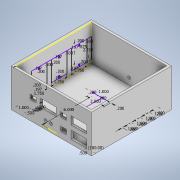
# Autodesk Inventor part: box thin walled
Saved by Autodesk Inventor 2020 (Build 240168000, 168)
## iProperties
Created: 2020-01-13
Part Number: box thin walled
Material: Generic
Document SubType Name: Modeling
Designer: ColinP
Density: 1 g/cm^3
Appearance: Default
Author: ColinP
Autodesk Inventor part; units mm, degrees
ref_plane "YZ Plane" through (0, 0, 0) normal (1, 0, 0) x (0, 1, 0)
ref_plane "XZ Plane" through (0, 0, 0) normal (0, 1, 0) x (-1, 0, 0)
ref_plane "XY Plane" through (0, 0, 0) normal (0, 0, 1) x (1, 0, 0)
sketch "Sketch1" plane through (0, 0, 0) normal (0, 1, 0) x (-1, 0, 0)
  line L0 (0, 0) -> (-114.3, 0)
  line L1 (-114.3, 0) -> (-114.3, -114.3)
  line L2 (-114.3, -114.3) -> (114.3, -114.3)
  line L3 (114.3, -114.3) -> (114.3, 114.3)
  line L4 (114.3, 114.3) -> (-114.3, 114.3)
  line L5 (-114.3, 114.3) -> (-114.3, 0)
  dimension "d0" = 114.3
  dimension "d1" = 114.3
  dimension "d2" = 228.6
  dimension "d3" = 228.6
  dimension "d4" = 90
  constraints: 12 end point, 4 perpendicular, 1 collinear, 1 horizontal, 1 point on line
  measures "d0" distance of L0.start L0.end
  measures "d1" distance of L0.end L1.end
  measures "d2" distance of L1.end L2.end
  measures "d3" distance of L2.end L3.end
  measures "d4" angle of L3 L2
extrude "Extrusion1" add sketch "Sketch1" along normal blind 6.35
sketch "Sketch3" plane through (0, 6.35, 0) normal (0, 1, 0) x (1, 0, 0)
  line L0 (114.3, 114.3) -> (-114.3, 114.3) projected
  line L1 (-114.3, 114.3) -> (-108.2442, 114.3)
  line L2 (-108.2442, 114.3) -> (-108.2442, -114.3)
  line L3 (-108.2442, 114.3) -> (120.3558, 114.3) construction
  line L4 (-108.2442, -114.3) -> (-108.2442, -107.95)
  line L5 (-108.2442, -107.95) -> (107.6558, -107.95)
  line L6 (107.6558, -107.95) -> (107.6558, 107.95)
  line L7 (107.6558, 107.95) -> (-108.2442, 107.95)
  line L8 (-114.3, 114.3) -> (-114.3, -114.3) projected
  line L9 (-114.3, -114.3) -> (114.3, -114.3) projected
  line L10 (114.3, -114.3) -> (114.3, 114.3) projected
  point P0 (0, 0)
  dimension "d19" = 228.6
  dimension "d20" = 90
  dimension "d21" = 6.35
  dimension "d22" = 215.9
  dimension "d23" = 215.9
  constraints: 14 end point, 4 perpendicular, 3 point on line, 1 horizontal, 1 vertical
  measures "d19" distance of L1.end L2.end
  measures "d20" angle of L2 L3
  measures "d21" distance of L2.end L4.end
  measures "d22" distance of L4.end L5.end
  measures "d23" distance of L5.end L6.end
extrude "Extrusion3" add sketch "Sketch3" along normal blind 101.6 contours L10 L9 L2 L5 L6 L7 L0 | L2 L9 L8 L0
sketch "Sketch4" plane through (-114.3, 0, 114.3) normal (0, 0, 1) x (1, 0, 0)
  line L0 (221.9558, 6.35) -> (221.9558, 107.95) projected
  line L1 (221.9558, 107.95) -> (221.9558, 44.45)
  line L2 (221.9558, 6.35) -> (6.0558, 6.35) projected
  line L3 (221.9558, 6.35) -> (221.9558, 12.7)
  line L4 (221.9558, 6.35) -> (221.9558, 107.95) projected
  line L5 (221.9558, 12.7) -> (215.6058, 12.7)
  line L6 (215.6058, 12.7) -> (215.6058, 35.2044)
  line L7 (215.6058, 35.2044) -> (170.597, 35.2044)
  line L8 (170.597, 35.2044) -> (170.597, 12.7)
  line L9 (170.597, 12.7) -> (215.6058, 12.7)
  line L10 (170.597, 12.7) -> (157.897, 12.7)
  line L11 (157.897, 12.7) -> (157.897, 35.2044)
  line L12 (157.897, 35.2044) -> (112.8882, 35.2044)
  line L13 (112.8882, 35.2044) -> (112.8882, 12.7)
  line L14 (112.8882, 12.7) -> (157.897, 12.7)
  line L15 (112.8882, 35.2044) -> (100.1882, 35.2044)
  line L16 (100.1882, 35.2044) -> (100.1882, 12.7)
  line L17 (100.1882, 12.7) -> (55.1794, 12.7)
  line L18 (55.1794, 12.7) -> (55.1794, 35.2044)
  line L19 (55.1794, 35.2044) -> (100.1882, 35.2044)
  line L20 (215.6058, 35.2044) -> (215.6058, 47.9044)
  line L21 (215.6058, 47.9044) -> (170.597, 47.9044)
  line L22 (170.597, 47.9044) -> (170.597, 70.4088)
  line L23 (170.597, 70.4088) -> (215.6058, 70.4088)
  line L24 (215.6058, 70.4088) -> (215.6058, 47.9044)
  line L25 (215.6058, 70.4088) -> (215.6058, 83.1088)
  point P0 (114.3, 0)
  point P1 (215.6058, 105.6132)
  point P2 (170.597, 105.6132)
  point P3 (170.597, 83.1088)
  dimension "d34" = 6.35
  dimension "d35" = 6.35
  dimension "d36" = 22.5044
  dimension "d37" = 45.0088
  dimension "d38" = 12.7
  dimension "d39" = 45.0088
  dimension "d40" = 12.7
  dimension "d41" = 45.0088
  dimension "d44" = 12.7
  dimension "d45" = 22.5044
  dimension "d46" = 12.7
  dimension "d47" = 22.5044
  constraints: 46 end point, 15 point on line, 14 perpendicular, 1 horizontal, 1 vertical
  measures "d34" distance of L0.start L3.end
  measures "d35" distance of L3.end L5.end
  measures "d36" distance of L5.end L6.end
  measures "d37" distance of L6.end L7.end
  measures "d38" distance of L8.end L10.end
  measures "d39" distance of L11.end L12.end
  measures "d40" distance of L12.end L15.end
  measures "d41" distance of L16.end L17.end
  measures "d44" distance of L6.end L20.end
  measures "d45" distance of L21.end L22.end
  measures "d46" distance of L23.end L25.end
  measures "d47" distance of L25.end point (215.606, 105.613)
sketch "Sketch9" plane through (-114.3, 0, 114.3) normal (0, 0, 1) x (1, 0, 0)
  line L0 (170.597, 47.9044) -> (170.597, 70.4088) projected
  line L1 (170.597, 70.4088) -> (170.597, 59.1566)
  line L2 (170.597, 59.1566) -> (157.897, 59.1566)
  line L3 (170.597, 35.0034) -> (170.597, 23.7512)
  line L4 (170.597, 23.7512) -> (157.897, 23.7512)
  line L5 (157.897, 59.1566) -> (157.897, 65.6066)
  line L6 (157.897, 65.6066) -> (141.197, 65.6066)
  line L7 (141.197, 65.6066) -> (141.197, 52.7034)
  line L8 (141.197, 52.7034) -> (157.897, 52.7034)
  line L9 (157.897, 52.7034) -> (157.897, 59.1566)
  line L10 (157.897, 23.7512) -> (157.897, 30.2012)
  line L11 (157.897, 30.2012) -> (141.197, 30.2012)
  line L12 (141.197, 30.2012) -> (141.197, 17.3012)
  line L13 (141.197, 17.3012) -> (157.897, 17.3012)
  line L14 (157.897, 17.3012) -> (157.897, 23.7512)
  point P0 (114.3, 0)
  point P1 (170.597, 105.6132)
  dimension "d64" = 11.2522
  dimension "d65" = 12.7
  dimension "d67" = 11.2522
  dimension "d68" = 12.7
  dimension "d82" = 6.45
  dimension "d83" = 12.9032
  dimension "d84" = 6.45
  dimension "d85" = 12.9
  constraints: 28 end point, 7 perpendicular, 4 point on line, 1 midpoint, 1 vertical
  measures "d64" distance of L0.end L1.end
  measures "d65" distance of L1.end L2.end
  measures "d67" distance of L3.start L3.end
  measures "d68" distance of L3.end L4.end
  measures "d82" distance of L2.end L5.end
  measures "d83" distance of L6.end L7.end
  measures "d84" distance of L4.end L10.end
  measures "d85" distance of L11.end L12.end
extrude "Extrusion4" cut sketch "Sketch4" against normal blind 114.3 contours L9 L8 L7 L6 | L21 L22 L23 L24
extrude "Extrusion6" cut sketch "Sketch9" against normal blind 114.3
sketch "Sketch14" plane through (-108.2442, 6.35, 107.95) normal (1, 0, 0) x (0, 0, -1)
  line L0 (215.9, 0) -> (0, 0) projected
  line L1 (0, 0) -> (0, 101.6) projected
  line L2 (-6.35, 101.6) -> (0, 101.6)
  line L3 (0, 101.6) -> (215.9, 101.6) projected
  line L4 (215.9, 0) -> (215.9, 101.6) projected
  line L5 (215.9, 66.675) -> (215.9, 9.525)
  line L6 (215.9, 66.675) -> (203.2, 66.675)
  line L7 (203.2, 66.675) -> (203.2, 9.525)
  line L8 (203.2, 9.525) -> (158.75, 9.525)
  line L9 (158.75, 9.525) -> (158.75, 66.675)
  line L10 (158.75, 66.675) -> (203.2, 66.675)
  line L11 (158.75, 66.675) -> (146.05, 66.675)
  line L12 (146.05, 66.675) -> (146.05, 9.525)
  line L13 (146.05, 9.525) -> (101.6, 9.525)
  line L14 (101.6, 9.525) -> (101.6, 66.675)
  line L15 (101.6, 66.675) -> (146.05, 66.675)
  line L16 (101.6, 66.675) -> (88.9, 66.675)
  line L17 (88.9, 66.675) -> (88.9, 9.525)
  line L18 (88.9, 9.525) -> (44.45, 9.525)
  line L19 (44.45, 9.525) -> (44.45, 66.675)
  line L20 (44.45, 66.675) -> (88.9, 66.675)
  line L21 (203.2, 66.675) -> (180.975, 66.675)
  line L22 (180.975, 66.675) -> (180.975, 61.675)
  line L23 (180.975, 9.525) -> (180.975, 14.525)
  circle A0 centre (180.975, 61.675) radius 2.54
  circle A1 centre (180.975, 14.525) radius 2.54
  line L24 (123.825, 66.675) -> (123.825, 61.675)
  line L25 (123.825, 9.525) -> (123.825, 14.525)
  circle A2 centre (123.825, 61.675) radius 2.54
  circle A3 centre (123.825, 14.525) radius 2.54
  line L26 (66.675, 66.675) -> (66.675, 61.675)
  line L27 (66.675, 9.525) -> (66.675, 14.525)
  circle A4 centre (66.675, 61.675) radius 2.54
  circle A5 centre (66.675, 14.525) radius 2.54
  point P0 (107.95, -6.35)
  dimension "d123" = 57.15
  dimension "d124" = 12.7
  dimension "d125" = 44.45
  dimension "d126" = 12.7
  dimension "d127" = 44.45
  dimension "d128" = 12.7
  dimension "d129" = 44.45
  dimension "d139" = 22.225
  dimension "d140" = 5
  dimension "d141" = 5
  dimension "d142" = 5.08
  dimension "d143" = 5.08
  dimension "d144" = 5
  dimension "d145" = 5
  dimension "d146" = 5.08
  dimension "d147" = 5.08
  dimension "d148" = 5
  dimension "d149" = 5
  dimension "d150" = 5.08
  dimension "d151" = 5.08
  constraints: 48 end point, 11 perpendicular, 11 point on line, 6 centre point, 6 coincident, 6 midpoint, 5 vertical, 1 collinear, 1 horizontal
  measures "d123" distance of L5.start L5.end
  measures "d124" distance of L5.start L6.end
  measures "d125" distance of L7.end L8.end
  measures "d126" distance of L9.end L11.end
  measures "d127" distance of L12.end L13.end
  measures "d128" distance of L14.end L16.end
  measures "d129" distance of L17.end L18.end
  measures "d139" distance of L6.end L21.end
  measures "d140" distance of L21.end L22.end
  measures "d141" distance of L23.start L23.end
  measures "d142" diameter of A0
  measures "d143" diameter of A1
  measures "d144" distance of L24.start L24.end
  measures "d145" distance of L25.start L25.end
  measures "d146" diameter of A2
  measures "d147" diameter of A3
  measures "d148" distance of L26.start L26.end
  measures "d149" distance of L27.start L27.end
  measures "d150" diameter of A4
  measures "d151" diameter of A5
sketch "Sketch15" plane through (-114.3, 0, 114.3) normal (0, 0, 1) x (1, 0, 0)
  line L0 (141.197, 65.6066) -> (141.197, 52.7034) projected
  line L1 (141.197, 59.155) -> (128.497, 59.155)
  line L2 (128.497, 59.155) -> (128.497, 70.4088)
  line L3 (128.497, 70.4088) -> (128.497, 47.9044)
  line L4 (215.6058, 47.9044) -> (170.597, 47.9044) projected
  line L5 (128.497, 47.9044) -> (83.4882, 47.9044)
  line L6 (83.4882, 47.9044) -> (83.4882, 70.4088)
  line L7 (83.4882, 70.4088) -> (128.497, 70.4088)
  line L8 (83.4882, 59.1566) -> (70.7882, 59.1566)
  line L9 (70.7882, 59.1566) -> (70.7882, 65.6066)
  line L10 (70.7882, 65.6066) -> (70.7882, 52.7034)
  line L11 (70.7882, 52.7034) -> (70.7882, 59.1566)
  line L12 (70.7882, 52.7034) -> (54.1004, 52.7034)
  line L13 (54.1004, 52.7034) -> (54.1004, 65.6066)
  line L14 (54.1004, 65.6066) -> (70.7882, 65.6066)
  point P0 (114.3, 0)
  dimension "d115" = 12.7
  dimension "d116" = 45.0088
  dimension "d117" = 12.7
  dimension "d118" = 16.6878
  constraints: 26 end point, 7 perpendicular, 4 horizontal, 2 midpoint, 2 point on line, 1 collinear
  measures "d115" distance of L1.start L1.end
  measures "d116" distance of L3.end L5.end
  measures "d117" distance of L8.start L8.end
  measures "d118" distance of L10.end L12.end
extrude "Extrusion9" cut sketch "Sketch15" against normal blind 114.3
sketch "Sketch16" plane through (-114.3, 0, 114.3) normal (0, 0, 1) x (1, 0, 0)
  line L0 (83.4882, 70.4088) -> (83.4882, 47.9044) projected
  line L1 (83.4882, 47.9044) -> (98.4911, 47.9044)
  line L2 (98.4911, 47.9044) -> (113.4941, 47.9044)
  line L3 (128.497, 47.9044) -> (83.4882, 47.9044) projected
  line L4 (113.4941, 47.9044) -> (128.497, 47.9044)
  line L5 (98.4911, 47.9044) -> (98.4911, 22.5044)
  line L6 (113.4941, 47.9044) -> (113.4941, 22.5044)
  circle A0 centre (98.4911, 22.5044) radius 4
  circle A1 centre (113.4941, 22.5044) radius 4
  point P0 (114.3, 0)
  dimension "d130" = 15.0029
  dimension "d131" = 15.0029
  dimension "d132" = 15.0029
  dimension "d133" = 25.4
  dimension "d134" = 25.4
  dimension "d135" = 8
  dimension "d136" = 8
  constraints: 10 end point, 2 centre point, 2 coincident, 2 vertical, 1 collinear, 1 horizontal, 1 point on line
  measures "d130" distance of L0.end L1.end
  measures "d131" distance of L1.end L2.end
  measures "d132" distance of L2.end L3.start
  measures "d133" distance of L1.end L5.end
  measures "d134" distance of L2.end L6.end
  measures "d135" diameter of A0
  measures "d136" diameter of A1
extrude "Extrusion10" cut sketch "Sketch16" against normal blind 76.2
sketch "Sketch17" plane through (0, 6.35, 0) normal (0, 1, 0) x (1, 0, 0)
  line L0 (107.6558, -107.95) -> (94.9558, -107.95)
  line L1 (107.6558, 107.95) -> (107.6558, -107.95) projected
  line L2 (107.6558, -107.95) -> (120.3558, -107.95) construction
  line L3 (94.9558, -6.35) -> (94.9558, 19.05)
  line L4 (94.9558, 19.05) -> (94.9558, 44.45)
  line L5 (94.9558, 44.45) -> (94.9558, 69.85)
  line L6 (94.9558, 69.85) -> (94.9558, 95.25)
  circle A0 centre (94.9558, -6.35) radius 2.54
  circle A1 centre (94.9558, 19.05) radius 2.54
  circle A2 centre (94.9558, 44.45) radius 2.54
  circle A3 centre (94.9558, 69.85) radius 2.54
  line L7 (-108.2442, -107.95) -> (-82.8442, -107.95)
  line L8 (107.6558, -107.95) -> (-108.2442, -107.95) projected
  line L9 (-82.8442, -107.95) -> (-82.8442, -95.25)
  line L10 (-82.8442, -95.25) -> (-82.8442, -82.55)
  line L11 (-82.8442, -82.55) -> (-82.8442, -69.85)
  circle A4 centre (-82.8442, -95.25) radius 2.54
  circle A5 centre (-82.8442, -82.55) radius 2.54
  circle A6 centre (-82.8442, -69.85) radius 2.54
  point P0 (0, 0)
  dimension "d152" = 12.7
  dimension "d153" = 180
  dimension "d159" = 25.4
  dimension "d161" = 25.4
  dimension "d162" = 25.4
  dimension "d163" = 25.4
  dimension "d164" = 5.08
  dimension "d165" = 5.08
  dimension "d166" = 5.08
  dimension "d167" = 5.08
  dimension "d173" = 25.4
  dimension "d174" = 12.7
  dimension "d175" = 12.7
  dimension "d176" = 12.7
  dimension "d177" = 5.08
  dimension "d178" = 5.08
  dimension "d179" = 5.08
  constraints: 20 end point, 7 centre point, 7 coincident, 6 point on line, 2 perpendicular, 1 collinear, 1 horizontal
  measures "d152" distance of L0.start L0.end
  measures "d153" angle of L0 L2
  measures "d159" distance of L3.start L3.end
  measures "d161" distance of L3.end L4.end
  measures "d162" distance of L4.end L5.end
  measures "d163" distance of L5.end L6.end
  measures "d164" diameter of A0
  measures "d165" diameter of A1
  measures "d166" diameter of A2
  measures "d167" diameter of A3
  measures "d173" distance of L7.start L7.end
  measures "d174" distance of L7.end L9.end
  measures "d175" distance of L9.end L10.end
  measures "d176" distance of L10.end L11.end
  measures "d177" diameter of A4
  measures "d178" diameter of A5
  measures "d179" diameter of A6
sketch "Sketch18" plane through (0, 6.35, 0) normal (0, 1, 0) x (1, 0, 0)
  line L0 (-8.3074, -72.1776) -> (-8.3074, -114.3)
  line L1 (14.197, -114.3) -> (-30.8118, -114.3) projected
  line L2 (-8.3074, -114.3) -> (-8.3074, 38.1)
  line L3 (-8.3074, 38.1) -> (-33.7074, 38.1)
  line L4 (-33.7074, 38.1) -> (17.0926, 38.1)
  circle A0 centre (-33.7074, 38.1) radius 2.54
  circle A1 centre (-8.3074, 38.1) radius 2.54
  circle A2 centre (17.0926, 38.1) radius 2.54
  point P0 (0, 0)
  dimension "d180" = 152.4
  dimension "d181" = 25.4
  dimension "d182" = 50.8
  dimension "d183" = 5.08
  dimension "d184" = 5.08
  dimension "d185" = 5.08
  constraints: 8 end point, 3 centre point, 3 coincident, 2 point on line, 1 midpoint, 1 perpendicular
  measures "d180" distance of L0.end L2.end
  measures "d181" distance of L2.end L3.end
  measures "d182" distance of L3.end L4.end
  measures "d183" diameter of A0
  measures "d184" diameter of A1
  measures "d185" diameter of A2
sketch "Sketch19" plane through (107.6558, 6.35, -107.95) normal (-1, 0, 0) x (0, 0, 1)
  line L0 (215.9, 41.5544) -> (88.9, 41.5544)
  line L1 (88.9, 41.5544) -> (139.7, 41.5544)
  line L2 (215.9, 28.8544) -> (88.9, 28.8544)
  line L3 (88.9, 28.8544) -> (139.7, 28.8544)
  line L4 (139.7, 41.5544) -> (139.7, 28.8544)
  line L5 (88.9, 41.5544) -> (88.9, 28.8544)
  point P0 (107.95, -6.35)
  dimension "d186" = 127
  dimension "d187" = 50.8
  dimension "d188" = 127
  constraints: 12 end point, 2 horizontal, 2 point on line, 1 perpendicular
  measures "d186" distance of L0.start L0.end
  measures "d187" distance of L0.end L1.end
  measures "d188" distance of L2.start L2.end
extrude "Extrusion11" add sketch "Sketch19" along normal blind 50.8
sketch "Sketch21" plane through (114.3, 0, -114.3) normal (0, 0, -1) x (-1, 0, 0)
  line L0 (114.3, 0) -> (114.3, 25.4)
  arc A0 (114.3, 25.4) -> (46.4215, 144.8435) centre (-24.7297, 25.4) ccw
  circle A1 centre (114.3, 25.4) radius 2.54
  circle A2 centre (114.3, 25.4) radius 4
  dimension "d195" = 25.4
  dimension "d196" = 5.08
  dimension "d197" = 8
  constraints: 3 centre point, 2 coincident, 2 end point, 2 point on circle, 1 tangent, 1 vertical
  measures "d195" distance of L0.start L0.end
  measures "d196" diameter of A1
  measures "d197" diameter of A2
extrude "Extrusion13" cut sketch "Sketch21" against normal blind 50.8
body "Solid1"
